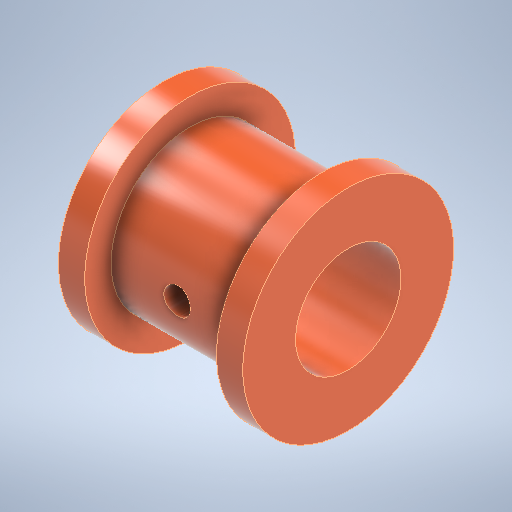
# Autodesk Inventor part: 146
Saved by Autodesk Inventor 2025.1 (Build 291241000, 241)
## iProperties
Created: 2024-08-05
Part Number: 146
Material: Rubber
Document SubType Name: Modeling
Designer: ffogue
Density: 0.93 g/cm^3
Appearance: Smooth - Light Orange
Author: ffogue
Autodesk Inventor part; units mm, degrees
ref_plane "YZ Plane" through (0, 0, 0) normal (1, 0, 0) x (0, 1, 0)
ref_plane "XY Plane" through (0, 0, 0) normal (0, 0, 1) x (1, 0, 0)
sketch "Sketch1" plane through (0, 0, 0) normal (0, 0, 1) x (1, 0, 0)
  line L0 (-7, 0) -> (-7, 8)
  line L1 (-7, 8) -> (-5, 8)
  line L2 (-5, 8) -> (-5, 6)
  line L3 (-5, 6) -> (5, 6)
  line L4 (5, 6) -> (5, 8)
  line L5 (5, 8) -> (7, 8)
  line L6 (7, 8) -> (7, 0)
  line L7 (7, 0) -> (-7, 0)
  point P0 (0, 0)
  point P1 (0, 0)
  dimension "d0" = 10
  dimension "d1" = 16
  dimension "d2" = 12
  dimension "d3" = 2
  dimension "d4" = 2
  dimension "d5" = 5
  constraints: 16 end point, 6 perpendicular, 2 point on line, 1 coincident, 1 midpoint, 1 vertical
  measures "d0" distance of L2.end L3.end
  measures "d1" diameter of L1 L7
  measures "d2" diameter of L3 L7
  measures "d3" distance of L0.end L1.end
  measures "d4" distance of L4.end L5.end
  measures "d5" distance from line of point (0, 0) L2
revolve "Revolution1" add sketch "Sketch1" angle 360 about axis through (7, 0, 0) along (-1, 0, 0)
ref_plane "Work Plane1" through (0, 6, 0) normal (0, 1, 0) x (-1, 0, 0)
sketch "Sketch3" plane through (0, 6, 0) normal (0, 1, 0) x (-1, 0, 0)
  point P0 (0, 0)
  point P1 (0, 0)
  constraints: 1 coincident
sketch "Sketch2" plane through (7, 0, 0) normal (1, 0, 0) x (0, 0, -1)
  circle A0 centre (0, 0) radius 8 projected
  point P0 (0, 0)
  constraints: 1 coincident
hole "Hole1" at (7, 0, 0) direction (-1, 0, 0) diameter 8 depth 14
hole "Hole2" at (0, 6, 0) direction (0, -1, 0) diameter 2 end through all
equation "\"d4\" = d3"
body "Solid1"
